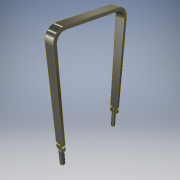
# Autodesk Inventor part: OAR3R010FLF_CurrentSense
Saved by Autodesk Inventor 2016 (Build 200138000, 138)
## iProperties
Created: 2016-09-07
Part Number: OAR3R010FLF_CurrentSense
Material: Generic
Document SubType Name: Modeling
Designer: jfixelle
Density: 1 g/cm^3
Appearance: Silver
Author: jfixelle
Autodesk Inventor part; units mm, degrees
ref_plane "YZ Plane" through (0, 0, 0) normal (1, 0, 0) x (0, 1, 0)
ref_plane "XZ Plane" through (0, 0, 0) normal (0, 1, 0) x (-1, 0, 0)
sketch "Sketch1" plane through (0, 0, 0) normal (0, 1, 0) x (-1, 0, 0)
  circle A0 centre (0, 7.62) radius 0.535
  point P0 (0, 0)
  dimension "d0" = 1.07
  dimension "d1" = 7.62
  constraints: 1 centre point
  measures "d0" diameter of A0
  measures "d1" distance of A0.centre point (0, 0)
extrude "Extrusion1" add sketch "Sketch1" along normal blind 3.94
ref_plane "Work Plane1" through (0, 0, 7.62) normal (0, 0, 1) x (1, 0, 0)
sketch "Sketch2" plane through (0, 0, 7.62) normal (0, 0, 1) x (1, 0, 0)
  line L0 (-0.95, 4.94) -> (0.95, 4.94)
  line L1 (0.95, 4.94) -> (0.95, 3.94)
  line L2 (0.95, 3.94) -> (-0.95, 3.94)
  line L3 (-0.95, 3.94) -> (-0.95, 4.94)
  line L4 (-0.535, 0) -> (0.535, 0) projected
  line L5 (0, 0) -> (0, -0.058)
  dimension "d5" = 3.94
  dimension "d6" = 1.9
  dimension "d7" = 0.95
  dimension "d8" = 1
  constraints: 10 end point, 2 parallel, 1 horizontal, 1 perpendicular, 1 vertical
  measures "d5" distance between parallel lines of L4 L2
  measures "d6" distance of L0.start L0.end
  measures "d7" distance between parallel lines of L3 L5
  measures "d8" distance of L0.end L1.end
extrude "Extrusion2" add sketch "Sketch2" along normal mid plane 0.6
fillet "Fillet1" radius 0.2 4 edges at (0.95, 3.94, 7.62) (0.95, 4.94, 7.62) (-0.95, 4.94, 7.62) (-0.95, 3.94, 7.62)
sketch "Sketch3" plane through (-0.75, 4.94, 7.92) normal (0, 1, 0) x (1, 0, 0)
  circle A0 centre (0.75, 0.3) radius 0.535
  point P0 (0.75, 7.92)
  dimension "d12" = 1.07
  dimension "d13" = 7.62
  constraints: 1 centre point
  measures "d12" diameter of A0
  measures "d13" distance of point (0.75, 7.92) A0.centre
extrude "Extrusion3" add sketch "Sketch3" along normal blind 0.6
sketch "Sketch4" plane through (0, 5.54, 7.62) normal (0, 1, 0) x (1, 0, 0)
  line L0 (0.75, 0.3) -> (0.95, 0.3) projected
  line L1 (-0.95, -0.3) -> (0.95, -0.3)
  line L2 (0.95, -0.3) -> (0.95, 0.3)
  line L3 (0.95, 0.3) -> (-0.95, 0.3)
  line L4 (-0.95, 0.3) -> (-0.95, -0.3)
  point P0 (0, 7.62)
  constraints: 8 end point, 2 parallel, 1 horizontal, 1 perpendicular
sketch "Sketch5" plane through (0, 0, 0) normal (1, 0, 0) x (0, 1, 0)
  line L0 (27.34, 0) -> (27.34, 5.62)
  line L1 (3.94, 7.085) -> (3.94, 7.32) projected
  line L2 (5.54, 7.085) -> (5.54, 8.155) projected
  line L3 (5.54, 7.62) -> (25.34, 7.62)
  arc A0 (27.34, 5.62) -> (25.34, 7.62) centre (25.34, 5.62) ccw
  point P0 (0, 0)
  dimension "d16" = 23.4
  dimension "d17" = 2
  constraints: 4 end point, 2 point on circle, 2 tangent, 1 centre point, 1 horizontal, 1 midpoint, 1 vertical
  measures "d16" distance between parallel lines of L1 L0
  measures "d17" radius of A0
sweep "Sweep1" add profiles "Sketch4" path "Sketch5" path curves L3 A0 L0
mirror "Mirror1" about plane through (0, 0, 0) normal (0, 0, 1) of "Sweep1", "Extrusion3", "Fillet1", "Extrusion2", "Extrusion1"
ref_plane "Work Plane2" through (0, 0, -7.62) normal (0, 0, 1) x (1, 0, 0)
body "Solid1"
